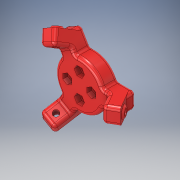
# Autodesk Inventor part: BottomPlatform
Saved by Autodesk Inventor 2019 (Build 230136000, 136)
## iProperties
Created: 2022-07-06
Part Number: BottomPlatform
Material: Generic
Document SubType Name: Modeling
Designer: zreik
Density: 1 g/cm^3
Appearance: Light Red
Author: zreik
Autodesk Inventor part; units mm, degrees
ref_plane "YZ Plane" through (0, 0, 0) normal (1, 0, 0) x (0, 1, 0)
ref_plane "XZ Plane" through (0, 0, 0) normal (0, 1, 0) x (-1, 0, 0)
ref_plane "XY Plane" through (0, 0, 0) normal (0, 0, 1) x (1, 0, 0)
sketch "Sketch1" plane through (0, 0, 0) normal (0, 0, 1) x (1, 0, 0)
  circle A0 centre (0, 0) radius 15
  line L0 (5, -5) -> (25, -5)
  line L1 (25, -5) -> (25, 5)
  line L2 (25, 5) -> (5, 5)
  line L3 (5, 5) -> (5, -5)
  line L4 (5, -5) -> (25, 5) construction
  line L5 (25, -5) -> (5, 5) construction
  point P0 (15, 0)
  dimension "d0" = 30
  dimension "d3" = 10
  dimension "d4" = 20
  dimension "d5" = 0
  constraints: 12 end point, 2 midpoint, 2 parallel, 1 coincident, 1 horizontal, 1 horizontal alignment, 1 perpendicular, 2 other
  measures "d3" distance of L0.end L1.end
  measures "d4" distance of L0.start L0.end
  measures "d5" vertical distance of point (0, 0) point (15, 0)
extrude "Extrusion1" add sketch "Sketch1" along normal mid plane 10 contours A0 L0 L3 L2 | L2 L3 L0 A0
extrude "Extrusion2" add sketch "Sketch1" along normal mid plane 10 contours A0 L0 L3 L2 | A0 L2 L1 L0 picked at (8.3333, 0)
chamfer "Chamfer1" distance 7 angle 30 1 edges at (25, 0, 5) measured on face at (0.1772, 3.8359, 5)
sketch "Sketch2" plane through (18, -5, 5) normal (0.5, 0, 0.8660254) x (0.8660254, 0, -0.5)
  line L0 (8.0829, 0) -> (0, 0)
  line L1 (0, 0) -> (0, 10)
  line L2 (0, 10) -> (8.0829, 10)
  line L3 (8.0829, 10) -> (8.0829, 0)
  line L4 (8.0829, 0) -> (0, 10) construction
  line L5 (0, 0) -> (8.0829, 10) construction
  line L6 (0, 10) -> (0, 0) projected
  line L7 (8.0829, 0) -> (8.0829, 10) projected
  line L8 (8.0829, 10) -> (0, 10) projected
  line L9 (0, 0) -> (8.0829, 0) projected
  point P0 (-13.0885, 5)
  point P1 (4.0415, 5)
  dimension "d11" = 0
  dimension "d12" = 0
  dimension "d13" = 0
  dimension "d14" = 0
  constraints: 12 end point, 2 midpoint, 2 parallel, 1 horizontal, 1 perpendicular
  measures "d11" distance between parallel lines of L1 L6
  measures "d12" distance between parallel lines of L7 L3
  measures "d13" distance between parallel lines of L8 L2
  measures "d14" distance between parallel lines of L9 L0
extrude "Extrusion3" add sketch "Sketch2" along normal blind 10
sketch "Sketch3" plane through (18, -5, 5) normal (-0.8660254, 0, 0.5) x (0.5, 0, 0.8660254)
  circle A0 centre (5, 5) radius 1.75
  line L0 (10, 10) -> (10, 0) projected
  line L1 (0, 10) -> (0, 0) projected
  line L2 (0, 0) -> (10, 0) projected
  line L3 (0, 10) -> (10, 10) projected
  point P0 (-13.3301, 5)
  dimension "d17" = 3.5
  dimension "d18" = 5
  dimension "d19" = 5
  dimension "d20" = 5
  dimension "d21" = 5
  constraints: 1 centre point
  measures "d17" diameter of A0
  measures "d18" distance from line of L0 A0.centre
  measures "d19" distance from line of L1 A0.centre
  measures "d20" distance from line of L2 A0.centre
  measures "d21" distance from line of L3 A0.centre
extrude "Extrusion8" cut sketch "Sketch3" against normal through all contours A0
sketch "Sketch6" plane through (25, -5, 0.9585) normal (0.8660254, 0, -0.5) x (-0.5, 0, -0.8660254)
  circle A0 centre (-5, 5) radius 3.5
  circle A1 centre (-5, 5) radius 1.75 projected
  point P0 (13.3301, 5)
  dimension "d40" = 7
  constraints: 1 centre point, 1 concentric
  measures "d40" diameter of A0
extrude "Extrusion9" add sketch "Sketch6" along normal blind 1.155
chamfer "Chamfer3" distance 1 angle 45 1 edges at (30.2503, 0, 7.7423)
pattern_circular "Circular Pattern1" count 3 over 360 about axis through (0, 0, 0) along (0, 0, 1) of "Extrusion3", "Extrusion2", "Chamfer1", "Extrusion8", "Chamfer3", "Extrusion9"
fillet "Fillet1" radius 2 9 edges at (25, 0, -5) (-12.5, 21.6506, -5) (-12.5, -21.6506, -5) (14.1421, 5, 0) (-2.7409, 14.7474, 0) (14.1421, -5, 0) (-2.7409, -14.7474, 0) (-11.4012, -9.7474, 0) (-11.4012, 9.7474, 0)
fillet "Fillet2" radius 2 3 edges at (-9, -15.5885, 5) (18, 0, 5) (-9, 15.5885, 5)
fillet "Fillet3" radius 2 3 edges at (-11.5, 19.9186, 13.6603) (23, 0, 13.6603) (-11.5, -19.9186, 13.6603)
fillet "Fillet4" radius 2 39 edges at (-15.9373, 17.6043, 12.8601) (-14.4745, 15.0705, 8.9641) (-13.2528, 12.9545, 5.2679) (-12.4144, 11.5024, 5) (-11.8106, 9.8172, 5) (-15, 0, 5) (-11.8106, -9.8172, 5) (-12.4144, -11.5024, 5) (-13.2528, -12.9545, 5.2679) (-14.4745, -15.0705, 8.9641) (-15.9373, -17.6043, 12.8601) (-18.0131, -21.1997, 11.1395) (-18.0131, 21.1997, 11.1395) (-9.3529, 26.1997, 11.1395) (-5.8142, 20.0705, 8.9641) (-4.5925, 17.9545, 5.2679) (-3.7542, 16.5024, 5) (-2.5967, 15.1369, 5) (7.5, 12.9904, 5) (14.4073, 5.3197, 5) (16.1686, 5, 5) (17.8453, 5, 5.2679) (20.2887, 5, 8.9641) (23.2144, 5, 12.8601) (27.366, 5, 11.1395) (-7.2771, 22.6043, 12.8601) (23.2144, -5, 12.8601) (20.2887, -5, 8.9641) (17.8453, -5, 5.2679) (16.1686, -5, 5) (14.4073, -5.3197, 5) (7.5, -12.9904, 5) (-2.5967, -15.1369, 5) (-3.7542, -16.5024, 5) (-4.5925, -17.9545, 5.2679) (-5.8142, -20.0705, 8.9641) (-7.2771, -22.6043, 12.8601) (-9.3529, -26.1997, 11.1395) (27.366, -5, 11.1395)
fillet "Fillet5" radius 2 27 edges at (-13.9531, -14.1675, -5) (-11.8106, -9.8172, -5) (-15, 0, -5) (-11.8106, 9.8172, -5) (-13.9531, 14.1675, -5) (-16.5372, 18.6433, -4.4142) (-16.8301, 19.1506, -1.0207) (-16.8301, -19.1506, -1.0207) (-16.5372, -18.6433, -4.4142) (-2.5967, -15.1369, -5) (-5.2929, -19.1675, -5) (-7.877, -23.6433, -4.4142) (-8.1699, -24.1506, -1.0207) (14.4073, -5.3197, -5) (19.246, -5, -5) (24.4142, -5, -4.4142) (25, -5, -1.0207) (7.5, -12.9904, -5) (14.4073, 5.3197, -5) (19.246, 5, -5) (24.4142, 5, -4.4142) (25, 5, -1.0207) (-2.5967, 15.1369, -5) (-5.2929, 19.1675, -5) (-7.877, 23.6433, -4.4142) (-8.1699, 24.1506, -1.0207) (7.5, 12.9904, -5)
sketch "Sketch7" plane through (0, 0, 5) normal (0, 0, 1) x (1, 0, 0)
  circle A0 centre (7.5, 0) radius 1.75
  line L0 (10.3, -1.6166) -> (7.5, -3.2332)
  line L1 (7.5, -3.2332) -> (4.7, -1.6166)
  line L2 (4.7, -1.6166) -> (4.7, 1.6166)
  line L3 (4.7, 1.6166) -> (7.5, 3.2332)
  line L4 (7.5, 3.2332) -> (10.3, 1.6166)
  line L5 (10.3, 1.6166) -> (10.3, -1.6166)
  line L6 (18.5774, -3) -> (18.5774, 3) projected
  point P0 (0, 0)
  dimension "d51" = 7.5
  dimension "d52" = 0
  dimension "d53" = 3.5
  dimension "d54" = 5.6
  constraints: 12 end point, 1 centre point, 1 coincident, 1 parallel, 13 other
  measures "d51" distance of A0.centre point (0, 0)
  measures "d52" vertical distance of point (0, 0) A0.centre
  measures "d53" diameter of A0
  measures "d54" distance between parallel lines of L2 L5
extrude "Extrusion10" cut sketch "Sketch7" against normal up to next contours A0
extrude "Extrusion11" cut sketch "Sketch7" against normal blind 3
pattern_circular "Circular Pattern2" count 4 over 360 about axis through (0, 0, 0) along (0, 0, 1) of "Extrusion11", "Extrusion10"
equation "\"d18\" = d19"
equation "\"d20\" = d21"
body "Solid1"
